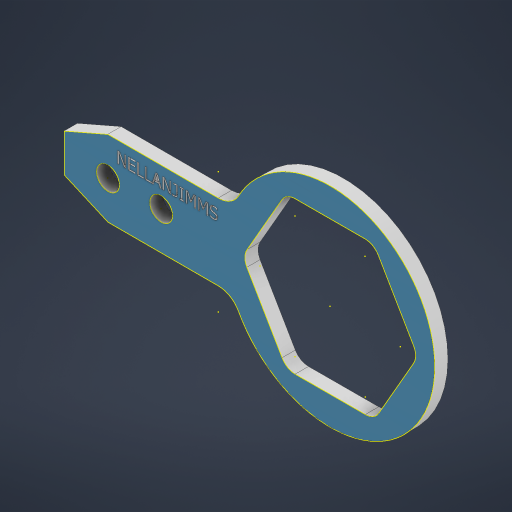
# Autodesk Inventor part: BICYCLE SPANNER
Saved by Autodesk Inventor 2023 (Build 270158000, 158)
## iProperties
Created: 2024-01-19
Part Number: BICYCLE SPANNER
Material: Generic
Document SubType Name: Modeling
Designer: User
Density: 1 g/cm^3
Appearance: Default
Author: User
Autodesk Inventor part; units mm, degrees
ref_plane "YZ Plane" through (0, 0, 0) normal (1, 0, 0) x (0, 1, 0)
ref_plane "XZ Plane" through (0, 0, 0) normal (0, 1, 0) x (-1, 0, 0)
ref_plane "XY Plane" through (0, 0, 0) normal (0, 0, 1) x (1, 0, 0)
sketch "Sketch1" plane through (0, 0, 0) normal (0, 0, 1) x (1, 0, 0)
  line L0 (25.3172, 36.0607) -> (43.8689, 4.105)
  line L1 (43.8881, -3.8949) -> (25.4895, -35.9391)
  line L2 (18.5709, -39.9557) -> (-18.3794, -40.0441)
  line L3 (-25.3172, -36.0607) -> (-43.8689, -4.105)
  line L4 (-43.8881, 3.8949) -> (-25.4895, 35.9391)
  line L5 (-18.5709, 39.9557) -> (18.3794, 40.0441)
  arc A0 (-48.3214, -26.2687) -> (-48.3214, 26.2687) centre (0, 0) ccw
  line L6 (-58.8643, 20) -> (-117, 20)
  line L7 (-58.8643, -20) -> (-117, -20)
  line L8 (-140, 10) -> (-140, -10)
  line L9 (-140, 0) -> (0, 0) construction
  line L10 (-117, 20) -> (-140, 10)
  line L11 (-140, -10) -> (-117, -20)
  arc A1 (-58.8643, 20) -> (-48.3214, 26.2687) centre (-58.8643, 32) ccw
  arc A2 (-48.3214, -26.2687) -> (-58.8643, -20) centre (-58.8643, -32) ccw
  arc A3 (-18.5709, 39.9557) -> (-25.4895, 35.9391) centre (-18.5518, 31.9557) ccw
  arc A4 (25.3172, 36.0607) -> (18.3794, 40.0441) centre (18.3985, 32.0441) ccw
  arc A5 (-43.8881, 3.8949) -> (-43.8689, -4.105) centre (-36.9503, -0.0885) ccw
  arc A6 (43.8881, -3.8949) -> (43.8689, 4.105) centre (36.9503, 0.0885) ccw
  arc A7 (18.5709, -39.9557) -> (25.4895, -35.9391) centre (18.5518, -31.9557) ccw
  arc A8 (-25.3172, -36.0607) -> (-18.3794, -40.0441) centre (-18.3985, -32.0441) ccw
  circle A9 centre (-117, 0) radius 6
  circle A10 centre (-89, 0) radius 6
  point P0 (22.9982, 40.0552)
  point P1 (46.1879, 0.1106)
  point P2 (23.1897, -39.9446)
  point P3 (-22.9982, -40.0552)
  point P4 (-46.1879, -0.1106)
  point P5 (-23.1897, 39.9446)
  point P6 (-0.0958, 39.9999)
  point P7 (0.0958, -39.9999)
  point P8 (-51.2348, -20)
  point P9 (-51.2348, 20)
  dimension "d1" = 79.9998
  dimension "d2" = 80
  dimension "d3" = 110
  dimension "d4" = 20
  dimension "d5" = 140
  dimension "d6" = 40
  dimension "d10" = 12
  dimension "d11" = 8
  dimension "d12" = 12
  dimension "d13" = 23
  dimension "d14" = 28
  constraints: 24 end point, 20 point on circle, 16 point on line, 16 tangent, 11 centre point, 7 equal radius, 3 horizontal, 3 midpoint, 2 coincident, 2 vertical alignment, 1 horizontal alignment, 1 vertical, 14 other
  measures "d1" vertical distance of point (-0.096, 40) point (0.096, -40)
  measures "d2" distance of point (46.188, 0.111) point (-22.998, -40.055)
  measures "d3" diameter of A0
  measures "d4" distance of L8.start L8.end
  measures "d5" distance of L9.start point (0, 0)
  measures "d6" distance between parallel lines of L7 L6
  measures "d10" radius of A1
  measures "d11" radius of A3
  measures "d12" diameter of A9
  measures "d13" horizontal distance of A9.centre L8.end
  measures "d14" distance of A10.centre A9.centre
extrude "Extrusion1" add sketch "Sketch1" along normal blind 7
sketch "Sketch2" plane through (0, 0, 7) normal (0, 0, 1) x (1, 0, 0)
  arc A0 (-48.3214, -26.2687) -> (-48.3214, 26.2687) centre (0, 0) ccw projected
  arc A1 (-58.8643, 20) -> (-48.3214, 26.2687) centre (-58.8643, 32) ccw projected
  line L0 (-58.8643, 20) -> (-117, 20) projected
  line L1 (-117, 20) -> (-140, 10) projected
  line L2 (-140, 10) -> (-140, -10) projected
  line L3 (-140, -10) -> (-117, -20) projected
  line L4 (-117, -20) -> (-58.8643, -20) projected
  arc A2 (-48.3214, -26.2687) -> (-58.8643, -20) centre (-58.8643, -32) ccw projected
  line L5 (-18.5709, 39.9557) -> (18.3794, 40.0441) projected
  arc A3 (25.3172, 36.0607) -> (18.3794, 40.0441) centre (18.3985, 32.0441) ccw projected
  line L6 (25.3172, 36.0607) -> (43.8689, 4.105) projected
  arc A4 (43.8881, -3.8949) -> (43.8689, 4.105) centre (36.9503, 0.0885) ccw projected
  line L7 (43.8881, -3.8949) -> (25.4895, -35.9391) projected
  arc A5 (18.5709, -39.9557) -> (25.4895, -35.9391) centre (18.5518, -31.9557) ccw projected
  line L8 (18.5709, -39.9557) -> (-18.3794, -40.0441) projected
  arc A6 (-25.3172, -36.0607) -> (-18.3794, -40.0441) centre (-18.3985, -32.0441) ccw projected
  line L9 (-25.3172, -36.0607) -> (-43.8689, -4.105) projected
  arc A7 (-43.8881, 3.8949) -> (-43.8689, -4.105) centre (-36.9503, -0.0885) ccw projected
  line L10 (-43.8881, 3.8949) -> (-25.4895, 35.9391) projected
  arc A8 (-18.5709, 39.9557) -> (-25.4895, 35.9391) centre (-18.5518, 31.9557) ccw projected
  circle A9 centre (-89, 0) radius 6 projected
  circle A10 centre (-117, 0) radius 6 projected
sketch "Sketch3" plane through (0, 0, 7) normal (0, 0, 1) x (1, 0, 0)
  line L0 (-112.4667, 15.3061) -> (-84.4197, 15.3061) construction
  line L1 (-84.4197, 15.3061) -> (-84.4197, 12.1494) construction
  line L2 (-84.4197, 12.1494) -> (-112.4667, 12.1494) construction
  line L3 (-112.4667, 12.1494) -> (-112.4667, 15.3061) construction
  line L4 (-107.4839, 9.0974) -> (-108.3935, 9.0974)
  line L5 (-108.3935, 9.0974) -> (-111.0925, 14.357)
  line L6 (-111.0925, 14.357) -> (-111.0925, 9.0974)
  line L7 (-111.0925, 9.0974) -> (-111.8488, 9.0974)
  line L8 (-111.8488, 9.0974) -> (-111.8488, 15.1974)
  line L9 (-111.8488, 15.1974) -> (-110.697, 15.1974)
  line L10 (-110.697, 15.1974) -> (-108.2402, 10.3678)
  line L11 (-108.2402, 10.3678) -> (-108.2402, 15.1974)
  line L12 (-108.2402, 15.1974) -> (-107.4839, 15.1974)
  line L13 (-107.4839, 15.1974) -> (-107.4839, 9.0974)
  line L14 (-106.2481, 9.0974) -> (-106.2481, 15.1974)
  line L15 (-106.2481, 15.1974) -> (-102.4319, 15.1974)
  line L16 (-102.4319, 15.1974) -> (-102.4319, 14.4757)
  line L17 (-102.4319, 14.4757) -> (-105.4374, 14.4757)
  line L18 (-105.4374, 14.4757) -> (-105.4374, 12.8048)
  line L19 (-105.4374, 12.8048) -> (-102.6345, 12.8048)
  line L20 (-102.6345, 12.8048) -> (-102.6345, 12.0831)
  line L21 (-102.6345, 12.0831) -> (-105.4374, 12.0831)
  line L22 (-105.4374, 12.0831) -> (-105.4374, 9.8191)
  line L23 (-105.4374, 9.8191) -> (-102.4319, 9.8191)
  line L24 (-102.4319, 9.8191) -> (-102.4319, 9.0974)
  line L25 (-102.4319, 9.0974) -> (-106.2481, 9.0974)
  line L26 (-98.0076, 9.0974) -> (-101.5421, 9.0974)
  line L27 (-101.5421, 9.0974) -> (-101.5421, 15.1974)
  line L28 (-101.5421, 15.1974) -> (-100.7314, 15.1974)
  line L29 (-100.7314, 15.1974) -> (-100.7314, 9.8191)
  line L30 (-100.7314, 9.8191) -> (-98.0076, 9.8191)
  line L31 (-98.0076, 9.8191) -> (-98.0076, 9.0974)
  line L32 (-93.8355, 9.0974) -> (-97.37, 9.0974)
  line L33 (-97.37, 9.0974) -> (-97.37, 15.1974)
  line L34 (-97.37, 15.1974) -> (-96.5593, 15.1974)
  line L35 (-96.5593, 15.1974) -> (-96.5593, 9.8191)
  line L36 (-96.5593, 9.8191) -> (-93.8355, 9.8191)
  line L37 (-93.8355, 9.8191) -> (-93.8355, 9.0974)
  line L38 (-93.8553, 9.0974) -> (-91.7989, 15.1974)
  line L39 (-91.7989, 15.1974) -> (-90.8003, 15.1974)
  line L40 (-90.8003, 15.1974) -> (-88.7439, 9.0974)
  line L41 (-88.7439, 9.0974) -> (-89.5991, 9.0974)
  line L42 (-89.5991, 9.0974) -> (-90.1528, 10.8028)
  line L43 (-90.1528, 10.8028) -> (-92.4811, 10.8028)
  line L44 (-92.4811, 10.8028) -> (-93.0347, 9.0974)
  line L45 (-93.0347, 9.0974) -> (-93.8553, 9.0974)
  line L46 (-90.3752, 11.4949) -> (-91.3194, 14.3669)
  line L47 (-91.3194, 14.3669) -> (-92.2586, 11.4949)
  line L48 (-92.2586, 11.4949) -> (-90.3752, 11.4949)
  line L49 (-83.8007, 9.0974) -> (-84.7102, 9.0974)
  line L50 (-84.7102, 9.0974) -> (-87.4093, 14.357)
  line L51 (-87.4093, 14.357) -> (-87.4093, 9.0974)
  line L52 (-87.4093, 9.0974) -> (-88.1656, 9.0974)
  line L53 (-88.1656, 9.0974) -> (-88.1656, 15.1974)
  line L54 (-88.1656, 15.1974) -> (-87.0138, 15.1974)
  line L55 (-87.0138, 15.1974) -> (-84.557, 10.3678)
  line L56 (-84.557, 10.3678) -> (-84.557, 15.1974)
  line L57 (-84.557, 15.1974) -> (-83.8007, 15.1974)
  line L58 (-83.8007, 15.1974) -> (-83.8007, 9.0974)
  spline S0 degree 2 poles (-80.2662, 10.6842) (-80.2662, 9.8833) (-81.245, 9.0133) (-82.0705, 9.0133) knots 0 0 0 1 2 2 2
  spline S1 degree 2 poles (-82.0705, 9.0133) (-82.2683, 9.0133) (-82.9257, 9.0825) (-83.1482, 9.132) knots 0 0 0 1 2 2 2
  line L59 (-83.1482, 9.132) -> (-83.1482, 9.913)
  line L60 (-83.1482, 9.913) -> (-83.1037, 9.913)
  spline S2 degree 2 poles (-83.1037, 9.913) (-82.9356, 9.8537) (-82.4363, 9.7153) (-82.1793, 9.7153) knots 0 0 0 1 2 2 2
  spline S3 degree 2 poles (-82.1793, 9.7153) (-81.8036, 9.7153) (-81.3538, 9.8883) (-81.2499, 10.0465) knots 0 0 0 1 2 2 2
  spline S4 degree 2 poles (-81.2499, 10.0465) (-81.1362, 10.2096) (-81.0769, 10.6842) (-81.0769, 10.9956) knots 0 0 0 1 2 2 2
  line L61 (-81.0769, 10.9956) -> (-81.0769, 14.5498)
  line L62 (-81.0769, 14.5498) -> (-82.3671, 14.5498)
  line L63 (-82.3671, 14.5498) -> (-82.3671, 15.1974)
  line L64 (-82.3671, 15.1974) -> (-80.2662, 15.1974)
  line L65 (-80.2662, 15.1974) -> (-80.2662, 10.6842)
  line L66 (-76.9444, 9.0974) -> (-79.3072, 9.0974)
  line L67 (-79.3072, 9.0974) -> (-79.3072, 9.7202)
  line L68 (-79.3072, 9.7202) -> (-78.5311, 9.7202)
  line L69 (-78.5311, 9.7202) -> (-78.5311, 14.5745)
  line L70 (-78.5311, 14.5745) -> (-79.3072, 14.5745)
  line L71 (-79.3072, 14.5745) -> (-79.3072, 15.1974)
  line L72 (-79.3072, 15.1974) -> (-76.9444, 15.1974)
  line L73 (-76.9444, 15.1974) -> (-76.9444, 14.5745)
  line L74 (-76.9444, 14.5745) -> (-77.7204, 14.5745)
  line L75 (-77.7204, 14.5745) -> (-77.7204, 9.7202)
  line L76 (-77.7204, 9.7202) -> (-76.9444, 9.7202)
  line L77 (-76.9444, 9.7202) -> (-76.9444, 9.0974)
  line L78 (-70.7109, 9.0974) -> (-71.5216, 9.0974)
  line L79 (-71.5216, 9.0974) -> (-71.5216, 14.3521)
  line L80 (-71.5216, 14.3521) -> (-73.1133, 10.7781)
  line L81 (-73.1133, 10.7781) -> (-73.6076, 10.7781)
  line L82 (-73.6076, 10.7781) -> (-75.1845, 14.3521)
  line L83 (-75.1845, 14.3521) -> (-75.1845, 9.0974)
  line L84 (-75.1845, 9.0974) -> (-75.9409, 9.0974)
  line L85 (-75.9409, 9.0974) -> (-75.9409, 15.1974)
  line L86 (-75.9409, 15.1974) -> (-74.8336, 15.1974)
  line L87 (-74.8336, 15.1974) -> (-73.311, 11.8013)
  line L88 (-73.311, 11.8013) -> (-71.8379, 15.1974)
  line L89 (-71.8379, 15.1974) -> (-70.7109, 15.1974)
  line L90 (-70.7109, 15.1974) -> (-70.7109, 9.0974)
  line L91 (-64.2451, 9.0974) -> (-65.0558, 9.0974)
  line L92 (-65.0558, 9.0974) -> (-65.0558, 14.3521)
  line L93 (-65.0558, 14.3521) -> (-66.6475, 10.7781)
  line L94 (-66.6475, 10.7781) -> (-67.1418, 10.7781)
  line L95 (-67.1418, 10.7781) -> (-68.7187, 14.3521)
  line L96 (-68.7187, 14.3521) -> (-68.7187, 9.0974)
  line L97 (-68.7187, 9.0974) -> (-69.4751, 9.0974)
  line L98 (-69.4751, 9.0974) -> (-69.4751, 15.1974)
  line L99 (-69.4751, 15.1974) -> (-68.3678, 15.1974)
  line L100 (-68.3678, 15.1974) -> (-66.8452, 11.8013)
  line L101 (-66.8452, 11.8013) -> (-65.3721, 15.1974)
  line L102 (-65.3721, 15.1974) -> (-64.2451, 15.1974)
  line L103 (-64.2451, 15.1974) -> (-64.2451, 9.0974)
  spline S5 degree 2 poles (-61.3088, 8.9886) (-61.9712, 8.9886) (-62.9005, 9.2654) (-63.3108, 9.4632) knots 0 0 0 1 2 2 2
  line L104 (-63.3108, 9.4632) -> (-63.3108, 10.4815)
  line L105 (-63.3108, 10.4815) -> (-63.2515, 10.4815)
  spline S6 degree 2 poles (-63.2515, 10.4815) (-62.8511, 10.1058) (-61.8377, 9.6906) (-61.3681, 9.6906) knots 0 0 0 1 2 2 2
  spline S7 degree 2 poles (-61.3681, 9.6906) (-60.6958, 9.6906) (-60.0087, 10.2492) (-60.0087, 10.7089) knots 0 0 0 1 2 2 2
  spline S8 degree 2 poles (-60.0087, 10.7089) (-60.0087, 11.0747) (-60.3696, 11.5295) (-60.7601, 11.6432) knots 0 0 0 1 2 2 2
  spline S9 degree 2 poles (-60.7601, 11.6432) (-61.0418, 11.7222) (-61.5114, 11.831) (-61.8624, 11.92) knots 0 0 0 1 2 2 2
  spline S10 degree 2 poles (-61.8624, 11.92) (-62.1788, 12.004) (-62.6781, 12.2561) (-62.8709, 12.4588) knots 0 0 0 1 2 2 2
  spline S11 degree 2 poles (-62.8709, 12.4588) (-63.0587, 12.6615) (-63.2663, 13.2052) (-63.2663, 13.5611) knots 0 0 0 1 2 2 2
  spline S12 degree 2 poles (-63.2663, 13.5611) (-63.2663, 14.3026) (-62.1096, 15.3061) (-61.2149, 15.3061) knots 0 0 0 1 2 2 2
  spline S13 degree 2 poles (-61.2149, 15.3061) (-60.7008, 15.3061) (-59.7912, 15.1034) (-59.4007, 14.9107) knots 0 0 0 1 2 2 2
  line L106 (-59.4007, 14.9107) -> (-59.4007, 13.9418)
  line L107 (-59.4007, 13.9418) -> (-59.46, 13.9418)
  spline S14 degree 2 poles (-59.46, 13.9418) (-59.7516, 14.2087) (-60.6612, 14.6042) (-61.1605, 14.6042) knots 0 0 0 1 2 2 2
  spline S15 degree 2 poles (-61.1605, 14.6042) (-61.724, 14.6042) (-62.421, 14.0752) (-62.421, 13.6452) knots 0 0 0 1 2 2 2
  spline S16 degree 2 poles (-62.421, 13.6452) (-62.421, 13.2596) (-62.0107, 12.7999) (-61.6251, 12.6961) knots 0 0 0 1 2 2 2
  spline S17 degree 2 poles (-61.6251, 12.6961) (-61.3681, 12.6269) (-60.6217, 12.4489) (-60.3745, 12.3748) knots 0 0 0 1 2 2 2
  spline S18 degree 2 poles (-60.3745, 12.3748) (-59.7467, 12.182) (-59.1634, 11.4059) (-59.1634, 10.8374) knots 0 0 0 1 2 2 2
  spline S19 degree 2 poles (-59.1634, 10.8374) (-59.1634, 10.4765) (-59.455, 9.7845) (-59.717, 9.5423) knots 0 0 0 1 2 2 2
  spline S20 degree 2 poles (-59.717, 9.5423) (-60.0087, 9.2753) (-60.7502, 8.9886) (-61.3088, 8.9886) knots 0 0 0 1 2 2 2
  point P0 (0, 0)
  constraints: 2 other
emboss "Emboss1" sketch "Sketch3" operation cut depth 2 direction (0, 0, -1)
body "Solid1"
